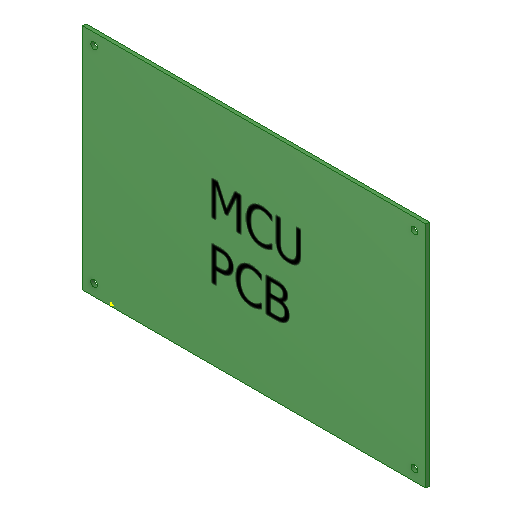
# Autodesk Inventor part: ASSEMBLY_Controller_PCB
Saved by Autodesk Inventor 2026.1 (Build 301233000, 233)
## iProperties
Created: 2018-08-02
Part Number: ASSEMBLY_Controller_PCB
Material: Generic
Document SubType Name: Modeling
Designer: Andrzej
Density: 1 g/cm^3
Appearance: Smooth - Dark Forest Green
Author: Andrzej
Autodesk Inventor part; units mm, degrees
ref_plane "YZ Plane" through (0, 0, 0) normal (1, 0, 0) x (0, 1, 0)
ref_plane "XZ Plane" through (0, 0, 0) normal (0, 1, 0) x (-1, 0, 0)
ref_plane "XY Plane" through (0, 0, 0) normal (0, 0, 1) x (1, 0, 0)
sketch "Sketch1" plane through (0, 0, 0) normal (0, 0, 1) x (1, 0, 0)
  line L0 (-12.6322, 98.9491) -> (137.3678, 98.9491)
  line L1 (137.3678, 98.9491) -> (137.3678, -1.0509)
  line L2 (137.3678, -1.0509) -> (-12.6322, -1.0509)
  line L3 (-12.6322, -1.0509) -> (-12.6322, 98.9491)
  point P0 (0, 0)
  point P1 (-7.6322, 93.9491)
  point P2 (132.3678, 93.9491)
  point P3 (132.3678, 3.9491)
  point P4 (-7.6322, 3.9491)
  dimension "d0" = 150
  dimension "d1" = 100
  dimension "d4" = 5
  dimension "d5" = 5
  dimension "d6" = 5
  dimension "d7" = 5
  constraints: 8 end point, 2 horizontal alignment, 2 parallel, 2 vertical alignment, 1 horizontal, 1 perpendicular
  measures "d0" distance of L1.end L2.end
  measures "d1" distance of L0.end L1.end
  measures "d4" distance from line of L3 point (-7.632, 93.949)
  measures "d5" distance from line of L1 point (132.368, 93.949)
  measures "d6" distance from line of L0 point (-7.632, 93.949)
  measures "d7" distance from line of L2 point (-7.632, 3.949)
extrude "Extrusion1" add sketch "Sketch1" along normal blind 1.5
sketch "Sketch2" plane through (0, 0, 1.5) normal (0, 0, 1) x (1, 0, 0)
  line L0 (42.2606, 69.8344) -> (131.918, 69.8344) construction
  line L1 (131.918, 69.8344) -> (131.918, 28.1713) construction
  line L2 (131.918, 28.1713) -> (42.2606, 28.1713) construction
  line L3 (42.2606, 28.1713) -> (42.2606, 69.8344) construction
  point P0 (0, 0)
  constraints: 2 other
hole "Hole1" at (132.3678, 3.9491, 0) at (132.3678, 93.9491, 0) at (-7.6322, 3.9491, 0) at (-7.6322, 93.9491, 0) direction (0, 0, 1) diameter 3 end through all
equation "\"d5\" = d4"
equation "\"d7\" = d6"
body "Solid1"
